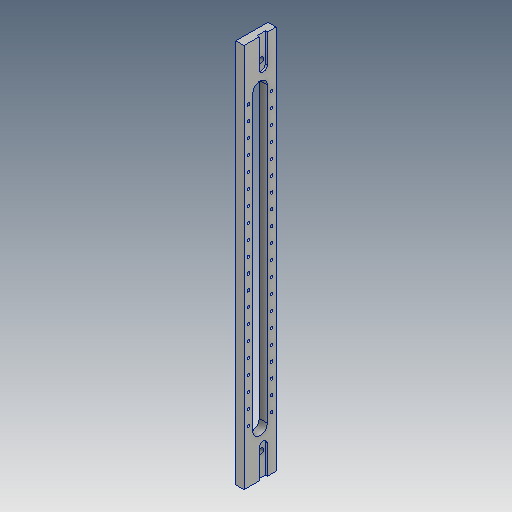
# Autodesk Inventor part: mppcMount
Saved by Autodesk Inventor 2018.2 (Build 222227000, 227)
## iProperties
Created: 2016-02-18
Part Number: mppcMount
Material: Aluminum 6061
Document SubType Name: Modeling
Designer: Sawaiz
Density: 2.7 g/cm^3
Appearance: Aluminum - Flat
Author: Sawaiz
Autodesk Inventor part; units mm, degrees
note: some values were not read from the file. Left out: dimensions or parameters whose unit could not be read.
ref_plane "YZ Plane" through (0, 0, 0) normal (1, 0, 0) x (0, 1, 0)
ref_plane "XZ Plane" through (0, 0, 0) normal (0, 1, 0) x (-1, 0, 0)
ref_plane "XY Plane" through (0, 0, 0) normal (0, 0, 1) x (1, 0, 0)
sketch "Sketch1" plane through (0, 0, 0) normal (0, 1, 0) x (-1, 0, 0)
  line L0 (-5.708, -114.16) -> (5.708, -114.16)
  line L1 (5.708, -114.16) -> (5.708, 114.16)
  line L2 (5.708, 114.16) -> (-5.708, 114.16)
  line L3 (-5.708, 114.16) -> (-5.708, -114.16)
  line L4 (-5.708, -114.16) -> (5.708, 114.16) construction
  line L5 (5.708, -114.16) -> (-5.708, 114.16) construction
  line L6 (-12.5, -150) -> (12.5, -150)
  line L7 (12.5, -150) -> (12.5, 150)
  line L8 (12.5, 150) -> (-12.5, 150)
  line L9 (-12.5, 150) -> (-12.5, -150)
  line L10 (-12.5, -150) -> (12.5, 150) construction
  line L11 (12.5, -150) -> (-12.5, 150) construction
  point P0 (0, 0)
  dimension "d0" = 11.416
  dimension "d1" = 228.32
  dimension "d2" = 300
  dimension "d3" = 25
  constraints: 24 end point, 4 midpoint, 4 parallel, 2 horizontal, 2 perpendicular
  measures "d0" distance of L1.end L2.end
  measures "d1" distance between parallel lines of L0 L2
  measures "d2" distance of L6.end L7.end
  measures "d3" distance of L7.end L8.end
extrude "Extrusion1" add sketch "Sketch1" along normal blind 6.35
sketch "Sketch2" plane through (0, 6.35, 0) normal (0, 1, 0) x (1, 0, 0)
  line L0 (5.708, 114.16) -> (5.708, -114.16) projected
  line L1 (5.708, -114.16) -> (-5.708, -114.16) projected
  line L2 (-5.708, -114.16) -> (-5.708, 114.16) projected
  line L3 (-5.708, 114.16) -> (5.708, 114.16) projected
  line L4 (12.5, 150) -> (-12.5, 150) projected
  line L5 (-12.5, 150) -> (-12.5, -150) projected
  line L6 (-12.5, -150) -> (12.5, -150) projected
  line L7 (12.5, -150) -> (12.5, 150) projected
  point P0 (0, 0)
  point P1 (-2.5, 132)
  dimension "d6" = 10
  dimension "d7" = 18
  measures "d6" distance from line of L5 point (-2.5, 132)
  measures "d7" distance from line of L4 point (-2.5, 132)
hole "Hole1" at (-2.5, 6.35, -132) direction (0, -1, 0) diameter 4.134 depth 14.2 tip angle 118 thread size "M5x0.8" class "6H" standard "ANSI Metric M Profile"
sketch "Sketch3" plane through (0, 6.35, 0) normal (0, 1, 0) x (1, 0, 0)
  circle A0 centre (-2.5, 132) radius 2.067 projected
  line L0 (5.708, 114.16) -> (5.708, -114.16) projected
  line L1 (5.708, -114.16) -> (-5.708, -114.16) projected
  line L2 (-5.708, -114.16) -> (-5.708, 114.16) projected
  line L3 (-5.708, 114.16) -> (5.708, 114.16) projected
  line L4 (12.5, 150) -> (-12.5, 150) projected
  line L5 (-12.5, 150) -> (-12.5, -150) projected
  line L6 (-12.5, -150) -> (12.5, -150) projected
  line L7 (12.5, -150) -> (12.5, 150) projected
  line L8 (0.675, 150) -> (-5.675, 150)
  line L9 (-5.675, 150) -> (-5.675, 124.6)
  line L10 (-5.675, 124.6) -> (0.675, 124.6)
  line L11 (0.675, 124.6) -> (0.675, 150)
  line L12 (-2.5, 124.6) -> (-2.5, 132) construction
  point P0 (0, 0)
  dimension "d15" = 6.35
  dimension "d16" = 25.4
  constraints: 10 end point, 2 parallel, 1 horizontal, 1 midpoint, 1 perpendicular, 1 point on line, 1 vertical
  measures "d15" distance of L9.end L10.end
  measures "d16" distance between parallel lines of L4 L10
extrude "Extrusion2" cut sketch "Sketch3" against normal blind 1.5875 contours L11 L10 L9 L4
fillet "Fillet1" radius 3.175 2 edges at (-5.675, 5.5562, -124.6) (0.675, 5.5562, -124.6)
mirror "Mirror1" about plane through (0, 0, 0) normal (0, 0, 1) of "Hole1", "Extrusion2", "Fillet1"
sketch "Sketch4" plane through (0, 0, 0) normal (0, -1, 0) x (1, 0, 0)
  circle A0 centre (-2.5, 132) radius 2.067 projected
  circle A1 centre (-2.5, -132) radius 2.067 projected
  line L0 (5.708, 114.16) -> (5.708, -114.16) projected
  line L1 (5.708, -114.16) -> (-5.708, -114.16) projected
  line L2 (-5.708, -114.16) -> (-5.708, 114.16) projected
  line L3 (-5.708, 114.16) -> (5.708, 114.16) projected
  line L4 (12.5, -150) -> (-12.5, -150) projected
  line L5 (12.5, 150) -> (12.5, -150) projected
  line L6 (-12.5, 150) -> (12.5, 150) projected
  line L7 (-12.5, -150) -> (-12.5, 150) projected
  arc A2 (5.708, 114.16) -> (-5.708, 114.16) centre (0, 114.16) ccw
  line L8 (-5.708, -114.16) -> (-5.708, 114.16) projected
  arc A3 (-5.708, -114.16) -> (5.708, -114.16) centre (0, -114.16) ccw
  point P0 (0, 0)
  constraints: 4 point on circle, 2 centre point, 2 tangent
extrude "Extrusion3" cut sketch "Sketch4" against normal through all contours L3 A2 | A3 L1
sketch "Sketch5" plane through (0, 0, 0) normal (0, -1, 0) x (1, 0, 0)
  line L0 (12.5, -150) -> (-12.5, -150) projected
  line L1 (12.5, 150) -> (12.5, -150) projected
  line L2 (-12.5, 150) -> (12.5, 150) projected
  line L3 (-12.5, -150) -> (-12.5, 150) projected
  arc A0 (5.708, 114.16) -> (-5.708, 114.16) centre (0, 114.16) ccw projected
  line L4 (5.708, 114.16) -> (5.708, -114.16) projected
  arc A1 (-5.708, -114.16) -> (5.708, -114.16) centre (0, -114.16) ccw projected
  line L5 (-5.708, -114.16) -> (-5.708, 114.16) projected
  circle A2 centre (-2.5, -132) radius 2.067 projected
  circle A3 centre (-2.5, 132) radius 2.067 projected
  point P0 (0, 0)
  point P1 (-9, -5.708)
  dimension "d22" = 9
  dimension "d23" = 5.708
  measures "d22" horizontal distance of point (0, 0) point (-9, -5.708)
  measures "d23" vertical distance of point (0, 0) point (-9, -5.708)
hole "Hole2" at (-9, 0, -5.708) direction (0, 1, 0) diameter 2.156 end through all thread size "4-40 UNC" class "2B" standard "ANSI Unified Screw Threads"
pattern_linear "Rectangular Pattern1" count 20 spacing 11.416 along (0, 0, 1) of "Hole2" first direction both ways yes
mirror "Mirror2" about plane through (0, 0, 0) normal (1, 0, 0) of "Hole2", "Rectangular Pattern1"
equation "\"d0\" = 2 * rubberizedCoating + ScintillatorWidth + 2 * silveringThickness"
equation "\"d1\" = 40 * silveringThickness + 20 * scintillatorWidth + 40 * rubberizedCoating"
equation "\"d2\" = width"
equation "\"d4\" = mppcMountThickness"
equation "\"d22\" = MountingScrewOffsett"
equation "\"d23\" = rubberizedCoating + 0.5 * ScintillatorThickness + silveringThickness"
equation "\"d33\" = 2 * silveringThickness + ScintillatorThickness + 2 * rubberizedCoating"
equation "\"silveringThickness\" = 0.2"
equation "\"mppcMountDepth\" = 6.35"
equation "\"MountingScrewOffsett\" = 9"
equation "\"opticalFiberDiameter\" = 1"
equation "\"opticalFiberClearence\" = 0.071"
equation "\"scintillatorEdgeClearence\" = 3"
equation "\"shallowTrackDepth\" = 1.142"
equation "\"deepTrackDepth\" = 5.571"
equation "\"fiberEdgeOffsett\" = 5"
equation "\"mppcMountThickness\" = 6.35"
equation "\"width\" = 300"
equation "\"facingGasketThickness\" = 1.5875"
equation "\"facingThickness\" = 12.7"
equation "\"ShallowTrackDepth\" = 1.142"
equation "\"ScintillatorEdgeClearence\" = 3"
equation "\"OpticalFiberClearence\" = 0.071"
equation "\"LoopLargeTrackRatio\" = 1.1"
equation "\"FiberEdgeOffsett\" = 5"
equation "\"FiberSensorClerence\" = 0.5"
equation "\"DeepTrackDepth\" = 5.571"
equation "\"ScintillatorWidth\" = 10"
equation "\"scintillatorWidth\" = 10"
equation "\"ScintillatorThickness\" = 10"
body "Solid1"
